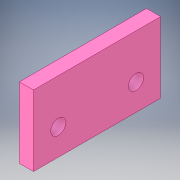
# Autodesk Inventor part: CHA_012_2inCrossSpacer
Saved by Autodesk Inventor 2018.3 (Build 223284000, 284)
## iProperties
Created: 2018-01-20
Part Number: CHA_012_2inCrossSpacer
Material: Aluminum 6061
Document SubType Name: Modeling
Designer: irodr
Density: 2.7 g/cm^3
Appearance: Pink
Mass: 29.8804 g
Surface Area: 48.8421 cm^2
Volume: 11.0668 cm^3
Author: irodr
Autodesk Inventor part; units mm, degrees
ref_plane "YZ Plane" through (0, 0, 0) normal (1, 0, 0) x (0, 1, 0)
ref_plane "XZ Plane" through (0, 0, 0) normal (0, 1, 0) x (-1, 0, 0)
ref_plane "XY Plane" through (0, 0, 0) normal (0, 0, 1) x (1, 0, 0)
sketch "Sketch1" plane through (0, 0, 0) normal (0, 0, 1) x (1, 0, 0)
  line L0 (0, 0) -> (6.35, 0)
  line L1 (6.35, 0) -> (6.35, 31.75)
  line L2 (6.35, 31.75) -> (0, 31.75)
  line L3 (0, 31.75) -> (0, 0)
  dimension "d0" = 6.35
  dimension "d1" = 31.75
  constraints: 8 end point, 2 parallel, 1 horizontal, 1 perpendicular
  measures "d0" distance of L2.end L1.end
  measures "d1" distance of L1.end L0.end
extrude "Extrusion1" add sketch "Sketch1" along normal blind 57.15
sketch "Sketch2" plane through (0, 0, 0) normal (-1, 0, 0) x (0, 0, 1)
  line L0 (0, 31.75) -> (0, 0) projected
  line L1 (0, 0) -> (57.15, 0) projected
  line L2 (57.15, 31.75) -> (57.15, 0) projected
  line L3 (0, 31.75) -> (57.15, 31.75) projected
  circle A0 centre (46.355, 1276.985) radius 2.3813 projected
  circle A1 centre (10.795, 1287.145) radius 2.3813 projected
  circle A2 centre (46.355, 1287.145) radius 2.3813 projected
  circle A3 centre (10.795, 1276.985) radius 2.3813 projected
  line L4 (53.975, 28.575) -> (3.175, 28.575) projected
  line L5 (53.975, 28.575) -> (53.975, 1292.225) projected
  line L6 (3.175, 1292.225) -> (53.975, 1292.225) projected
  line L7 (3.175, 28.575) -> (3.175, 1292.225) projected
  circle A4 centre (11.1125, 11.8745) radius 2.4892 projected
  circle A5 centre (46.0375, 11.8745) radius 2.4892 projected
  constraints: 2 coincident, 1 other
hole "Hole1" at (0, 11.8745, 11.1125) at (0, 11.8745, 46.0375) direction (1, 0, 0) diameter 6.7564 end through all
body "Solid1"
